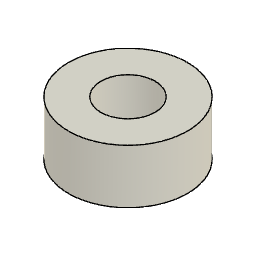
オムニ2024-Complete v4 (Autodesk Fusion 360 archive; units mm, degrees)
design "シリコンチューブ"
Autodesk Fusion 360 part; units mm, degrees
sketch "スケッチ1" plane through (0, 0, 0) normal (0, 0, 1) x (1, 0, 0)
  circle A0 centre (0, 0) radius 5.5
  circle A1 centre (0, 0) radius 2.5
  dimension "d1" = 11
  dimension "d2" = 5
  constraint coincident A0.centre A1.centre
  measures "d1" diameter of A0
  measures "d2" diameter of A1
extrude "押し出し1" add sketch "スケッチ1" along normal blind 5

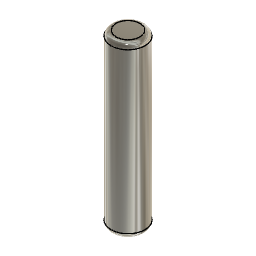
design "棒"
Autodesk Fusion 360 part; units mm, degrees
sketch "スケッチ1" plane through (0, 0, 0) normal (0, 0, 1) x (1, 0, 0)
  circle A0 centre (0, 0) radius 1
  dimension "d1" = 2
  constraint coincident A0.centre origin
  measures "d1" diameter of A0
extrude "押し出し1" add sketch "スケッチ1" along normal blind 10
fillet "フィレット1" radius 0.3 2 edges at (-0.9323, -0.3616, 10) (-0.9323, -0.3616, 0)

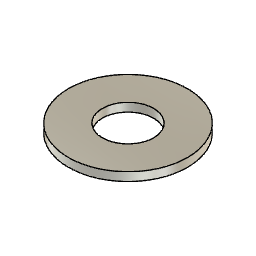
design "ワッシャー　小"
Autodesk Fusion 360 part; units mm, degrees
sketch "スケッチ1" plane through (0, 0, 0) normal (0, 0, 1) x (1, 0, 0)
  circle A0 centre (0, 0) radius 1.5
  circle A1 centre (0, 0) radius 3.5
  dimension "d1" = 3
  dimension "d2" = 7
  constraint coincident A0.centre A1.centre
  measures "d1" diameter of A0
  measures "d2" diameter of A1
extrude "押し出し1" add sketch "スケッチ1" along normal blind 0.5

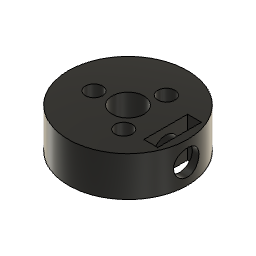
design "オムニ2024-3"
Autodesk Fusion 360 part; units mm, degrees
sketch "スケッチ1" plane through (0, 0, 0) normal (0, 0, 1) x (1, 0, 0)
  circle A0 centre (0, 0) radius 7.5
  dimension "d1" = 15
  constraint coincident A0.centre origin
  measures "d1" diameter of A0
extrude "押し出し1" add sketch "スケッチ1" along normal blind 5
sketch "スケッチ2" plane through (0, 0, 5) normal (0, 0, 1) x (-1, 0, 0)
  circle A0 centre (0, 0) radius 7.5
  circle A1 centre (0, 0) radius 2
  dimension "d4" = 4
  constraint coincident A0.centre A1.centre
  measures "d4" diameter of A1
extrude "押し出し2" cut sketch "スケッチ2" against normal blind 18 contours A1
sketch "スケッチ3" plane through (0, 0, -15) normal (0, 0, 1) x (-1, 0, 0)
  circle A0 centre (-1.3364, -3.4921) radius 1.075
  circle A1 centre (3.6924, 0.5887) radius 1.075
  circle A2 centre (-2.3561, 2.9034) radius 1.075
  circle A3 centre (0, 0) radius 2
  arc A4 (6.9441, -2.8337) -> (7.4957, 0.253) centre (0, 0) ccw
  line L0 (7.4957, 0.253) -> (3.5477, 3.5514)
  arc A5 (3.8294, 4.4336) -> (3.5477, 3.5514) centre (3.8682, 3.9351) ccw
  line L1 (3.8294, 4.4336) -> (5.9261, 4.5969)
  arc A6 (5.9261, 4.5969) -> (3.5288, 6.618) centre (0, 0) ccw
  line L2 (3.5288, 6.618) -> (-1.3018, 4.8481)
  arc A7 (-1.9249, 5.5332) -> (-1.3018, 4.8481) centre (-1.4738, 5.3176) ccw
  line L3 (-1.9249, 5.5332) -> (-1.0179, 7.4306)
  arc A8 (-1.0179, 7.4306) -> (-3.967, 6.365) centre (0, 0) ccw
  line L4 (-3.967, 6.365) -> (-4.8495, 1.2966)
  arc A9 (-5.7543, 1.0996) -> (-4.8495, 1.2966) centre (-5.342, 1.3824) ccw
  line L5 (-5.7543, 1.0996) -> (-6.9441, 2.8337)
  arc A10 (-6.9441, 2.8337) -> (-7.4957, -0.253) centre (0, 0) ccw
  line L6 (-7.4957, -0.253) -> (-3.5477, -3.5514)
  arc A11 (-3.8294, -4.4336) -> (-3.5477, -3.5514) centre (-3.8682, -3.9351) ccw
  line L7 (-3.8294, -4.4336) -> (-5.9261, -4.5969)
  arc A12 (-5.9261, -4.5969) -> (-3.5288, -6.618) centre (0, 0) ccw
  line L8 (-3.5288, -6.618) -> (1.7202, -4.6948)
  arc A13 (1.7202, -4.6948) -> (2.5, -4.3301) centre (0, 0) ccw
  line L9 (2.5, -4.3301) -> (1.0179, -7.4306)
  arc A14 (1.0179, -7.4306) -> (3.967, -6.365) centre (0, 0) ccw
  line L10 (3.967, -6.365) -> (4.8495, -1.2966)
  arc A15 (5.7543, -1.0996) -> (4.8495, -1.2966) centre (5.342, -1.3824) ccw
  line L11 (5.7543, -1.0996) -> (6.9441, -2.8337)
extrude "押し出し3" cut sketch "スケッチ3" along normal blind 28 contours A0 | A1 | A2
sketch "スケッチ4" plane through (0, 0, 0) normal (1, 0, 0) x (0, 1, 0)
  circle A0 centre (0, 2.5) radius 1.6
  dimension "d9" = 3.2
  measures "d9" diameter of A0
extrude "押し出し4" cut sketch "スケッチ4" along normal blind 10
sketch "スケッチ5" plane through (0, 0, 5) normal (0, 0, 1) x (-1, 0, 0)
  circle A0 centre (-1.3364, -3.4921) radius 1.075
  circle A1 centre (3.6924, 0.5887) radius 1.075
  circle A2 centre (-2.3561, 2.9034) radius 1.075
  circle A3 centre (0, 0) radius 2
  circle A4 centre (0, 0) radius 7.5
  line L0 (-4.75, 0) -> (-4.75, 2.75)
  line L1 (-4.75, 2.75) -> (-6.5, 2.75)
  line L2 (-6.5, 2.75) -> (-6.5, 0)
  line L3 (-6.5, -2.75) -> (-6.5, 0)
  line L4 (-4.75, 0) -> (-4.75, -2.75)
  line L5 (-4.75, -2.75) -> (-6.5, -2.75)
  dimension "d12" = 1.75
  dimension "d13" = 2.75
  constraint vertical L0
  constraint horizontal L1
  constraint vertical L2
  measures "d12" distance of L2.end L0.start
  measures "d13" distance of L2.end L1.end
extrude "押し出し5" cut sketch "スケッチ5" against normal blind 9 contours L0 L1 L2 L3 L4 L5

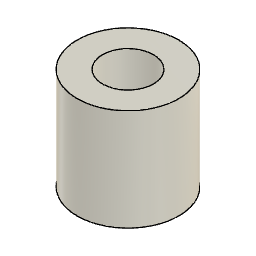
design "プラスチックスペーサー"
Autodesk Fusion 360 part; units mm, degrees
sketch "スケッチ1" plane through (0, 0, 0) normal (0, 0, 1) x (1, 0, 0)
  circle A0 centre (0, 0) radius 2.5
  circle A1 centre (0, 0) radius 1.25
  dimension "d1" = 5
  dimension "d2" = 2.5
  constraint coincident A0.centre A1.centre
  constraint concentric A0 A1
  measures "d1" diameter of A0
  measures "d2" diameter of A1
extrude "押し出し1" add sketch "スケッチ1" along normal blind 5

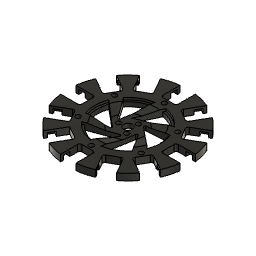
design "オムニ2024-1"
Autodesk Fusion 360 part; units mm, degrees
sketch "スケッチ2" plane through (0, 0, 0) normal (0, 0, 1) x (1, 0, 0)
  circle A0 centre (0, 0) radius 27.5
  line L0 (-3.5, 18.5) -> (3.5, 18.5)
  line L1 (3.5, 18.5) -> (3.5, 30.5)
  line L2 (3.5, 30.5) -> (-3.5, 30.5)
  line L3 (-3.5, 30.5) -> (-3.5, 18.5)
  line L4 (-18.2811, 24.6638) -> (-12.2811, 14.2715)
  line L5 (-6.2189, 17.7715) -> (-12.2189, 28.1638)
  line L6 (-12.2811, 14.2715) -> (-6.2189, 17.7715)
  line L7 (-12.2189, 28.1638) -> (-18.2811, 24.6638)
  line L8 (-28.1638, 12.2189) -> (-17.7715, 6.2189)
  line L9 (-14.2715, 12.2811) -> (-24.6638, 18.2811)
  line L10 (-17.7715, 6.2189) -> (-14.2715, 12.2811)
  line L11 (-24.6638, 18.2811) -> (-28.1638, 12.2189)
  line L12 (-30.5, -3.5) -> (-18.5, -3.5)
  line L13 (-18.5, 3.5) -> (-30.5, 3.5)
  line L14 (-18.5, -3.5) -> (-18.5, 3.5)
  line L15 (-30.5, 3.5) -> (-30.5, -3.5)
  line L16 (-24.6638, -18.2811) -> (-14.2715, -12.2811)
  line L17 (-17.7715, -6.2189) -> (-28.1638, -12.2189)
  line L18 (-14.2715, -12.2811) -> (-17.7715, -6.2189)
  line L19 (-28.1638, -12.2189) -> (-24.6638, -18.2811)
  line L20 (-12.2189, -28.1638) -> (-6.2189, -17.7715)
  line L21 (-12.2811, -14.2715) -> (-18.2811, -24.6638)
  line L22 (-6.2189, -17.7715) -> (-12.2811, -14.2715)
  line L23 (-18.2811, -24.6638) -> (-12.2189, -28.1638)
  line L24 (3.5, -30.5) -> (3.5, -18.5)
  line L25 (-3.5, -18.5) -> (-3.5, -30.5)
  line L26 (3.5, -18.5) -> (-3.5, -18.5)
  line L27 (-3.5, -30.5) -> (3.5, -30.5)
  line L28 (18.2811, -24.6638) -> (12.2811, -14.2715)
  line L29 (6.2189, -17.7715) -> (12.2189, -28.1638)
  line L30 (12.2811, -14.2715) -> (6.2189, -17.7715)
  line L31 (12.2189, -28.1638) -> (18.2811, -24.6638)
  line L32 (28.1638, -12.2189) -> (17.7715, -6.2189)
  line L33 (14.2715, -12.2811) -> (24.6638, -18.2811)
  line L34 (17.7715, -6.2189) -> (14.2715, -12.2811)
  line L35 (24.6638, -18.2811) -> (28.1638, -12.2189)
  line L36 (30.5, 3.5) -> (18.5, 3.5)
  line L37 (18.5, -3.5) -> (30.5, -3.5)
  line L38 (18.5, 3.5) -> (18.5, -3.5)
  line L39 (30.5, -3.5) -> (30.5, 3.5)
  line L40 (24.6638, 18.2811) -> (14.2715, 12.2811)
  line L41 (17.7715, 6.2189) -> (28.1638, 12.2189)
  line L42 (14.2715, 12.2811) -> (17.7715, 6.2189)
  line L43 (28.1638, 12.2189) -> (24.6638, 18.2811)
  line L44 (12.2189, 28.1638) -> (6.2189, 17.7715)
  line L45 (12.2811, 14.2715) -> (18.2811, 24.6638)
  line L46 (6.2189, 17.7715) -> (12.2811, 14.2715)
  line L47 (18.2811, 24.6638) -> (12.2189, 28.1638)
  dimension "d2" = 55
  dimension "d4" = 360
  constraint coincident A0.centre origin
  constraint horizontal L0
  constraint vertical L1
  constraint horizontal L2
  constraint vertical L3
  measures "d2" diameter of A0
extrude "押し出し1" add sketch "スケッチ2" along normal blind 3 contours A0 L0 L1 L3 L4 L5 L6 L8 L9 L10 L12 L13 L14 L16 L17 L18 L20 L21 L22 L24 L25 L26 L28 L29 L30 L32 L33 L34 L36 L37 L38 L40 L41 L42 L44 L45 L46
sketch "スケッチ3" plane through (0, 0, 3) normal (0, 0, 1) x (-1, 0, 0)
  arc A0 (-10.6071, -25.372) -> (-3.5, -27.2764) centre (0, 0) ccw
  line L0 (-3.5, -27.2764) -> (-3.5, -18.5)
  line L1 (-3.5, -18.5) -> (3.5, -18.5)
  line L2 (3.5, -18.5) -> (3.5, -27.2764)
  arc A1 (3.5, -27.2764) -> (10.6071, -25.372) centre (0, 0) ccw
  line L3 (10.6071, -25.372) -> (6.2189, -17.7715)
  line L4 (6.2189, -17.7715) -> (12.2811, -14.2715)
  line L5 (12.2811, -14.2715) -> (16.6693, -21.872)
  arc A2 (16.6693, -21.872) -> (21.872, -16.6693) centre (0, 0) ccw
  line L6 (21.872, -16.6693) -> (14.2715, -12.2811)
  line L7 (14.2715, -12.2811) -> (17.7715, -6.2189)
  line L8 (17.7715, -6.2189) -> (25.372, -10.6071)
  arc A3 (25.372, -10.6071) -> (27.2764, -3.5) centre (0, 0) ccw
  line L9 (27.2764, -3.5) -> (18.5, -3.5)
  line L10 (18.5, -3.5) -> (18.5, 3.5)
  line L11 (18.5, 3.5) -> (27.2764, 3.5)
  arc A4 (27.2764, 3.5) -> (25.372, 10.6071) centre (0, 0) ccw
  line L12 (25.372, 10.6071) -> (17.7715, 6.2189)
  line L13 (17.7715, 6.2189) -> (14.2715, 12.2811)
  line L14 (14.2715, 12.2811) -> (21.872, 16.6693)
  arc A5 (21.872, 16.6693) -> (16.6693, 21.872) centre (0, 0) ccw
  line L15 (16.6693, 21.872) -> (12.2811, 14.2715)
  line L16 (12.2811, 14.2715) -> (6.2189, 17.7715)
  line L17 (6.2189, 17.7715) -> (10.6071, 25.372)
  arc A6 (10.6071, 25.372) -> (3.5, 27.2764) centre (0, 0) ccw
  line L18 (3.5, 27.2764) -> (3.5, 18.5)
  line L19 (3.5, 18.5) -> (-3.5, 18.5)
  line L20 (-3.5, 18.5) -> (-3.5, 27.2764)
  arc A7 (-3.5, 27.2764) -> (-10.6071, 25.372) centre (0, 0) ccw
  line L21 (-10.6071, 25.372) -> (-6.2189, 17.7715)
  line L22 (-6.2189, 17.7715) -> (-12.2811, 14.2715)
  line L23 (-12.2811, 14.2715) -> (-16.6693, 21.872)
  arc A8 (-16.6693, 21.872) -> (-21.872, 16.6693) centre (0, 0) ccw
  line L24 (-21.872, 16.6693) -> (-14.2715, 12.2811)
  line L25 (-14.2715, 12.2811) -> (-17.7715, 6.2189)
  line L26 (-17.7715, 6.2189) -> (-25.372, 10.6071)
  arc A9 (-25.372, 10.6071) -> (-27.2764, 3.5) centre (0, 0) ccw
  line L27 (-27.2764, 3.5) -> (-18.5, 3.5)
  line L28 (-18.5, 3.5) -> (-18.5, -3.5)
  line L29 (-18.5, -3.5) -> (-27.2764, -3.5)
  arc A10 (-27.2764, -3.5) -> (-25.372, -10.6071) centre (0, 0) ccw
  line L30 (-25.372, -10.6071) -> (-17.7715, -6.2189)
  line L31 (-17.7715, -6.2189) -> (-14.2715, -12.2811)
  line L32 (-14.2715, -12.2811) -> (-21.872, -16.6693)
  arc A11 (-21.872, -16.6693) -> (-16.6693, -21.872) centre (0, 0) ccw
  line L33 (-16.6693, -21.872) -> (-12.2811, -14.2715)
  line L34 (-12.2811, -14.2715) -> (-6.2189, -17.7715)
  line L35 (-6.2189, -17.7715) -> (-10.6071, -25.372)
  circle A12 centre (0, 0) radius 15
  circle A13 centre (0, 0) radius 2
  circle A14 centre (0, 0) radius 5
  line L36 (2.5, -14.7902) -> (4.9259, -0.8577)
  line L37 (-2.5, -14.7902) -> (2.5, -4.3301)
  line L38 (14.0587, -5.23) -> (3.2057, 3.8371)
  line L39 (11.5587, -9.5602) -> (5, 0)
  line L40 (11.5587, 9.5602) -> (-1.7202, 4.6948)
  line L41 (14.0587, 5.23) -> (2.5, 4.3301)
  line L42 (-2.5, 14.7902) -> (-4.9259, 0.8577)
  line L43 (2.5, 14.7902) -> (-2.5, 4.3301)
  line L44 (-14.0587, 5.23) -> (-3.2057, -3.8371)
  line L45 (-11.5587, 9.5602) -> (-5, 0)
  line L46 (-11.5587, -9.5602) -> (1.7202, -4.6948)
  line L47 (-14.0587, -5.23) -> (-2.5, -4.3301)
  dimension "d8" = 360
  constraint coincident A0.centre A1.centre
  constraint concentric A12 A14
  constraint coincident A12 L36.start
  constraint coincident A14 L36.end
  constraint tangent A14 L36
  constraint coincident A12 L37.start
  constraint coincident A14 L37.end
extrude "押し出し2" cut sketch "スケッチ3" against normal blind 30 contours A12 A14 L38 L41 | A12 A14 L40 L43 | A12 A14 L36 L39 | A12 A14 L42 L45 | A12 A14 L37 L46 | A12 A14 L44 L47 | A13
sketch "スケッチ4" plane through (0, 0, 0) normal (0, 1, 0) x (1, 0, 0)
  line L0 (0, -6) -> (0, -2)
  line L1 (0, -2) -> (10, -3)
  line L2 (10, -3) -> (10, -7)
  line L3 (10, -7) -> (0, -6)
  constraint vertical L0
  constraint parallel L0 L2
sketch "スケッチ5" plane through (0, 0, 0) normal (0, 0, 1) x (1, 0, 0)
  circle A0 centre (0, 0) radius 15
  circle A1 centre (0, 0) radius 14
  constraint coincident A0.centre A1.centre
extrude "押し出し3" add sketch "スケッチ5" along normal blind 2
sketch "スケッチ6" plane through (0, 0, 0) normal (0, 0, -1) x (1, 0, 0)
  line L0 (-13.0187, 5.1491) -> (-2.5, 4.3301)
  arc A0 (-2.5, 4.3301) -> (-3.2057, 3.8371) centre (0, 0) ccw
  line L1 (-3.2057, 3.8371) -> (-13.241, -4.5469)
  arc A1 (-13.0187, 5.1491) -> (-13.241, -4.5469) centre (0, 0) ccw
  line L2 (-10.9686, -8.7) -> (-5, 0)
  arc A2 (-5, 0) -> (-4.9259, -0.8577) centre (0, 0) ccw
  line L3 (-4.9259, -0.8577) -> (-2.6828, -13.7406)
  arc A3 (-10.9686, -8.7) -> (-2.6828, -13.7406) centre (0, 0) ccw
  line L4 (2.0501, -13.8491) -> (-2.5, -4.3301)
  arc A4 (-2.5, -4.3301) -> (-1.7202, -4.6948) centre (0, 0) ccw
  line L5 (-1.7202, -4.6948) -> (10.5583, -9.1936)
  arc A5 (2.0501, -13.8491) -> (10.5583, -9.1936) centre (0, 0) ccw
  arc A6 (-2.0501, 13.8491) -> (-10.5583, 9.1936) centre (0, 0) ccw
  line L6 (-2.0501, 13.8491) -> (2.5, 4.3301)
  arc A7 (2.5, 4.3301) -> (1.7202, 4.6948) centre (0, 0) ccw
  line L7 (1.7202, 4.6948) -> (-10.5583, 9.1936)
  arc A8 (10.9686, 8.7) -> (2.6828, 13.7406) centre (0, 0) ccw
  line L8 (10.9686, 8.7) -> (5, 0)
  arc A9 (5, 0) -> (4.9259, 0.8577) centre (0, 0) ccw
  line L9 (4.9259, 0.8577) -> (2.6828, 13.7406)
  circle A10 centre (0, 0) radius 2
  arc A11 (13.0187, -5.1491) -> (13.241, 4.5469) centre (0, 0) ccw
  line L10 (13.0187, -5.1491) -> (2.5, -4.3301)
  arc A12 (2.5, -4.3301) -> (3.2057, -3.8371) centre (0, 0) ccw
  line L11 (3.2057, -3.8371) -> (13.241, 4.5469)
  arc A13 (3.5, -27.2764) -> (10.6071, -25.372) centre (0, 0) ccw
  line L12 (10.6071, -25.372) -> (6.2189, -17.7715)
  line L13 (6.2189, -17.7715) -> (12.2811, -14.2715)
  line L14 (12.2811, -14.2715) -> (16.6693, -21.872)
  arc A14 (16.6693, -21.872) -> (21.872, -16.6693) centre (0, 0) ccw
  line L15 (21.872, -16.6693) -> (14.2715, -12.2811)
  line L16 (14.2715, -12.2811) -> (17.7715, -6.2189)
  line L17 (17.7715, -6.2189) -> (25.372, -10.6071)
  arc A15 (25.372, -10.6071) -> (27.2764, -3.5) centre (0, 0) ccw
  line L18 (27.2764, -3.5) -> (18.5, -3.5)
  line L19 (18.5, -3.5) -> (18.5, 3.5)
  line L20 (18.5, 3.5) -> (27.2764, 3.5)
  arc A16 (27.2764, 3.5) -> (25.372, 10.6071) centre (0, 0) ccw
  line L21 (25.372, 10.6071) -> (17.7715, 6.2189)
  line L22 (17.7715, 6.2189) -> (14.2715, 12.2811)
  line L23 (14.2715, 12.2811) -> (21.872, 16.6693)
  arc A17 (21.872, 16.6693) -> (16.6693, 21.872) centre (0, 0) ccw
  line L24 (16.6693, 21.872) -> (12.2811, 14.2715)
  line L25 (12.2811, 14.2715) -> (6.2189, 17.7715)
  line L26 (6.2189, 17.7715) -> (10.6071, 25.372)
  arc A18 (10.6071, 25.372) -> (3.5, 27.2764) centre (0, 0) ccw
  line L27 (3.5, 27.2764) -> (3.5, 18.5)
  line L28 (3.5, 18.5) -> (-3.5, 18.5)
  line L29 (-3.5, 18.5) -> (-3.5, 27.2764)
  arc A19 (-3.5, 27.2764) -> (-10.6071, 25.372) centre (0, 0) ccw
  line L30 (-10.6071, 25.372) -> (-6.2189, 17.7715)
  line L31 (-6.2189, 17.7715) -> (-12.2811, 14.2715)
  line L32 (-12.2811, 14.2715) -> (-16.6693, 21.872)
  arc A20 (-16.6693, 21.872) -> (-21.872, 16.6693) centre (0, 0) ccw
  line L33 (-21.872, 16.6693) -> (-14.2715, 12.2811)
  line L34 (-14.2715, 12.2811) -> (-17.7715, 6.2189)
  line L35 (-17.7715, 6.2189) -> (-25.372, 10.6071)
  arc A21 (-25.372, 10.6071) -> (-27.2764, 3.5) centre (0, 0) ccw
  line L36 (-27.2764, 3.5) -> (-18.5, 3.5)
  line L37 (-18.5, 3.5) -> (-18.5, -3.5)
  line L38 (-18.5, -3.5) -> (-27.2764, -3.5)
  arc A22 (-27.2764, -3.5) -> (-25.372, -10.6071) centre (0, 0) ccw
  line L39 (-25.372, -10.6071) -> (-17.7715, -6.2189)
  line L40 (-17.7715, -6.2189) -> (-14.2715, -12.2811)
  line L41 (-14.2715, -12.2811) -> (-21.872, -16.6693)
  arc A23 (-21.872, -16.6693) -> (-16.6693, -21.872) centre (0, 0) ccw
  line L42 (-16.6693, -21.872) -> (-12.2811, -14.2715)
  line L43 (-12.2811, -14.2715) -> (-6.2189, -17.7715)
  line L44 (-6.2189, -17.7715) -> (-10.6071, -25.372)
  arc A24 (-10.6071, -25.372) -> (-3.5, -27.2764) centre (0, 0) ccw
  line L45 (-3.5, -27.2764) -> (-3.5, -18.5)
  line L46 (-3.5, -18.5) -> (3.5, -18.5)
  line L47 (3.5, -18.5) -> (3.5, -27.2764)
  line L48 (5.4, -26) -> (0, -26)
  line L49 (0, -23) -> (5.4, -23)
  line L50 (5.4, -23) -> (5.4, -26)
  line L51 (0, -23) -> (-5.4, -23)
  line L52 (-5.4, -23) -> (-5.4, -26)
  line L53 (-5.4, -26) -> (0, -26)
  line L54 (11.5, -19.9186) -> (6.8235, -22.6186)
  line L55 (6.8235, -22.6186) -> (8.3235, -25.2167)
  line L56 (8.3235, -25.2167) -> (13, -22.5167)
  line L57 (17.6765, -19.8167) -> (13, -22.5167)
  line L58 (11.5, -19.9186) -> (16.1765, -17.2186)
  line L59 (16.1765, -17.2186) -> (17.6765, -19.8167)
  line L60 (19.9186, -11.5) -> (17.2186, -16.1765)
  line L61 (17.2186, -16.1765) -> (19.8167, -17.6765)
  line L62 (19.8167, -17.6765) -> (22.5167, -13)
  line L63 (25.2167, -8.3235) -> (22.5167, -13)
  line L64 (19.9186, -11.5) -> (22.6186, -6.8235)
  line L65 (22.6186, -6.8235) -> (25.2167, -8.3235)
  line L66 (23, 0) -> (23, -5.4)
  line L67 (23, -5.4) -> (26, -5.4)
  line L68 (26, -5.4) -> (26, 0)
  line L69 (26, 5.4) -> (26, 0)
  line L70 (23, 0) -> (23, 5.4)
  line L71 (23, 5.4) -> (26, 5.4)
  line L72 (19.9186, 11.5) -> (22.6186, 6.8235)
  line L73 (22.6186, 6.8235) -> (25.2167, 8.3235)
  line L74 (25.2167, 8.3235) -> (22.5167, 13)
  line L75 (19.8167, 17.6765) -> (22.5167, 13)
  line L76 (19.9186, 11.5) -> (17.2186, 16.1765)
  line L77 (17.2186, 16.1765) -> (19.8167, 17.6765)
  line L78 (11.5, 19.9186) -> (16.1765, 17.2186)
  line L79 (16.1765, 17.2186) -> (17.6765, 19.8167)
  line L80 (17.6765, 19.8167) -> (13, 22.5167)
  line L81 (8.3235, 25.2167) -> (13, 22.5167)
  line L82 (11.5, 19.9186) -> (6.8235, 22.6186)
  line L83 (6.8235, 22.6186) -> (8.3235, 25.2167)
  line L84 (0, 23) -> (5.4, 23)
  line L85 (5.4, 23) -> (5.4, 26)
  line L86 (5.4, 26) -> (0, 26)
  line L87 (-5.4, 26) -> (0, 26)
  line L88 (0, 23) -> (-5.4, 23)
  line L89 (-5.4, 23) -> (-5.4, 26)
  line L90 (-11.5, 19.9186) -> (-6.8235, 22.6186)
  line L91 (-6.8235, 22.6186) -> (-8.3235, 25.2167)
  line L92 (-8.3235, 25.2167) -> (-13, 22.5167)
  line L93 (-17.6765, 19.8167) -> (-13, 22.5167)
  line L94 (-11.5, 19.9186) -> (-16.1765, 17.2186)
  line L95 (-16.1765, 17.2186) -> (-17.6765, 19.8167)
  line L96 (-19.9186, 11.5) -> (-17.2186, 16.1765)
  line L97 (-17.2186, 16.1765) -> (-19.8167, 17.6765)
  line L98 (-19.8167, 17.6765) -> (-22.5167, 13)
  line L99 (-25.2167, 8.3235) -> (-22.5167, 13)
  line L100 (-19.9186, 11.5) -> (-22.6186, 6.8235)
  line L101 (-22.6186, 6.8235) -> (-25.2167, 8.3235)
  line L102 (-23, 0) -> (-23, 5.4)
  line L103 (-23, 5.4) -> (-26, 5.4)
  line L104 (-26, 5.4) -> (-26, 0)
  line L105 (-26, -5.4) -> (-26, 0)
  line L106 (-23, 0) -> (-23, -5.4)
  line L107 (-23, -5.4) -> (-26, -5.4)
  line L108 (-19.9186, -11.5) -> (-22.6186, -6.8235)
  line L109 (-22.6186, -6.8235) -> (-25.2167, -8.3235)
  line L110 (-25.2167, -8.3235) -> (-22.5167, -13)
  line L111 (-19.8167, -17.6765) -> (-22.5167, -13)
  line L112 (-19.9186, -11.5) -> (-17.2186, -16.1765)
  line L113 (-17.2186, -16.1765) -> (-19.8167, -17.6765)
  line L114 (-11.5, -19.9186) -> (-16.1765, -17.2186)
  line L115 (-16.1765, -17.2186) -> (-17.6765, -19.8167)
  line L116 (-17.6765, -19.8167) -> (-13, -22.5167)
  line L117 (-8.3235, -25.2167) -> (-13, -22.5167)
  line L118 (-11.5, -19.9186) -> (-6.8235, -22.6186)
  line L119 (-6.8235, -22.6186) -> (-8.3235, -25.2167)
  dimension "d15" = 360
  constraint horizontal L48
  constraint horizontal L49
  constraint vertical L50
extrude "押し出し4" cut sketch "スケッチ6" against normal blind 2 contours L47 L48 L49 L50 | L12 L54 L55 L56 | L45 L51 L52 L53 | L14 L57 L58 L59 | L44 L117 L118 L119 | L15 L60 L61 L62 | L42 L114 L115 L116 | L17 L63 L64 L65 | L41 L111 L112 L113 | L18 L66 L67 L68 | L39 L108 L109 L110 | L20 L69 L70 L71 | L38 L105 L106 L107 | L21 L72 L73 L74 | L36 L102 L103 L104 | L23 L75 L76 L77 | L35 L99 L100 L101 | L24 L78 L79 L80 | L33 L96 L97 L98 | L26 L81 L82 L83 | L32 L93 L94 L95 | L27 L84 L85 L86 | L30 L90 L91 L92 | L29 L87 L88 L89
sketch "スケッチ7" plane through (0, 0, 3) normal (0, 0, 1) x (-1, 0, 0)
  line L0 (-2.5, 4.3301) -> (2.5, 14.7902)
  arc A0 (11.5587, 9.5602) -> (2.5, 14.7902) centre (0, 0) ccw
  line L1 (11.5587, 9.5602) -> (-1.7202, 4.6948)
  arc A1 (-1.7202, 4.6948) -> (-2.5, 4.3301) centre (0, 0) ccw
  line L2 (5, 0) -> (11.5587, -9.5602)
  arc A2 (2.5, -14.7902) -> (11.5587, -9.5602) centre (0, 0) ccw
  line L3 (2.5, -14.7902) -> (4.9259, -0.8577)
  arc A3 (4.9259, -0.8577) -> (5, 0) centre (0, 0) ccw
  line L4 (-5, 0) -> (-11.5587, 9.5602)
  arc A4 (-2.5, 14.7902) -> (-11.5587, 9.5602) centre (0, 0) ccw
  line L5 (-2.5, 14.7902) -> (-4.9259, 0.8577)
  arc A5 (-4.9259, 0.8577) -> (-5, 0) centre (0, 0) ccw
  line L6 (2.5, 4.3301) -> (14.0587, 5.23)
  arc A6 (14.0587, -5.23) -> (14.0587, 5.23) centre (0, 0) ccw
  line L7 (14.0587, -5.23) -> (3.2057, 3.8371)
  arc A7 (3.2057, 3.8371) -> (2.5, 4.3301) centre (0, 0) ccw
  arc A8 (1.7202, -4.6948) -> (2.5, -4.3301) centre (0, 0) ccw
  line L8 (2.5, -4.3301) -> (-2.5, -14.7902)
  arc A9 (-11.5587, -9.5602) -> (-2.5, -14.7902) centre (0, 0) ccw
  line L9 (-11.5587, -9.5602) -> (1.7202, -4.6948)
  line L10 (-2.5, -4.3301) -> (-14.0587, -5.23)
  arc A10 (-14.0587, 5.23) -> (-14.0587, -5.23) centre (0, 0) ccw
  line L11 (-14.0587, 5.23) -> (-3.2057, -3.8371)
  arc A11 (-3.2057, -3.8371) -> (-2.5, -4.3301) centre (0, 0) ccw
  circle A12 centre (0, 0) radius 2
  arc A13 (-10.6071, -25.372) -> (-3.5, -27.2764) centre (0, 0) ccw
  line L12 (-3.5, -27.2764) -> (-3.5, -18.5)
  line L13 (-3.5, -18.5) -> (3.5, -18.5)
  line L14 (3.5, -18.5) -> (3.5, -27.2764)
  arc A14 (3.5, -27.2764) -> (10.6071, -25.372) centre (0, 0) ccw
  line L15 (10.6071, -25.372) -> (6.2189, -17.7715)
  line L16 (6.2189, -17.7715) -> (12.2811, -14.2715)
  line L17 (12.2811, -14.2715) -> (16.6693, -21.872)
  arc A15 (16.6693, -21.872) -> (21.872, -16.6693) centre (0, 0) ccw
  line L18 (21.872, -16.6693) -> (14.2715, -12.2811)
  line L19 (14.2715, -12.2811) -> (17.7715, -6.2189)
  line L20 (17.7715, -6.2189) -> (25.372, -10.6071)
  arc A16 (25.372, -10.6071) -> (27.2764, -3.5) centre (0, 0) ccw
  line L21 (27.2764, -3.5) -> (18.5, -3.5)
  line L22 (18.5, -3.5) -> (18.5, 3.5)
  line L23 (18.5, 3.5) -> (27.2764, 3.5)
  arc A17 (27.2764, 3.5) -> (25.372, 10.6071) centre (0, 0) ccw
  line L24 (25.372, 10.6071) -> (17.7715, 6.2189)
  line L25 (17.7715, 6.2189) -> (14.2715, 12.2811)
  line L26 (14.2715, 12.2811) -> (21.872, 16.6693)
  arc A18 (21.872, 16.6693) -> (16.6693, 21.872) centre (0, 0) ccw
  line L27 (16.6693, 21.872) -> (12.2811, 14.2715)
  line L28 (12.2811, 14.2715) -> (6.2189, 17.7715)
  line L29 (6.2189, 17.7715) -> (10.6071, 25.372)
  arc A19 (10.6071, 25.372) -> (3.5, 27.2764) centre (0, 0) ccw
  line L30 (3.5, 27.2764) -> (3.5, 18.5)
  line L31 (3.5, 18.5) -> (-3.5, 18.5)
  line L32 (-3.5, 18.5) -> (-3.5, 27.2764)
  arc A20 (-3.5, 27.2764) -> (-10.6071, 25.372) centre (0, 0) ccw
  line L33 (-10.6071, 25.372) -> (-6.2189, 17.7715)
  line L34 (-6.2189, 17.7715) -> (-12.2811, 14.2715)
  line L35 (-12.2811, 14.2715) -> (-16.6693, 21.872)
  arc A21 (-16.6693, 21.872) -> (-21.872, 16.6693) centre (0, 0) ccw
  line L36 (-21.872, 16.6693) -> (-14.2715, 12.2811)
  line L37 (-14.2715, 12.2811) -> (-17.7715, 6.2189)
  line L38 (-17.7715, 6.2189) -> (-25.372, 10.6071)
  arc A22 (-25.372, 10.6071) -> (-27.2764, 3.5) centre (0, 0) ccw
  line L39 (-27.2764, 3.5) -> (-18.5, 3.5)
  line L40 (-18.5, 3.5) -> (-18.5, -3.5)
  line L41 (-18.5, -3.5) -> (-27.2764, -3.5)
  arc A23 (-27.2764, -3.5) -> (-25.372, -10.6071) centre (0, 0) ccw
  line L42 (-25.372, -10.6071) -> (-17.7715, -6.2189)
  line L43 (-17.7715, -6.2189) -> (-14.2715, -12.2811)
  line L44 (-14.2715, -12.2811) -> (-21.872, -16.6693)
  arc A24 (-21.872, -16.6693) -> (-16.6693, -21.872) centre (0, 0) ccw
  line L45 (-16.6693, -21.872) -> (-12.2811, -14.2715)
  line L46 (-12.2811, -14.2715) -> (-6.2189, -17.7715)
  line L47 (-6.2189, -17.7715) -> (-10.6071, -25.372)
  circle A25 centre (0, 0) radius 7.5
  dimension "d18" = 15
  constraint concentric A0 A25
  measures "d18" diameter of A25
extrude "押し出し5" cut sketch "スケッチ7" against normal blind 1 contours L0 L1 A1 L2 L3 A3 L4 L5 A5 L6 L7 A7 A8 L8 L9 L10 L11 A11 A25
sketch "スケッチ8" plane through (0, 0, 0) normal (0, 1, 0) x (1, 0, 0)
  line L0 (0, -10) -> (-7.5, -10)
  line L1 (0, -10) -> (0, -2)
  line L2 (0, -2) -> (-7.5, -2)
  line L3 (-7.5, -2) -> (-13, -3)
  line L4 (-13, -3) -> (-8, -10)
  line L5 (-8, -10) -> (-7.5, -10)
  dimension "d21" = 7.5
  dimension "d22" = 7.5
  constraint horizontal L0
  constraint perpendicular L0 L1
  constraint perpendicular L1 L2
  constraint parallel L0 L5
  measures "d21" distance of L0.start L0.end
  measures "d22" distance of L1.end L2.end
revolve "回転2" cut sketch "スケッチ8" angle 360 about axis through (0, 0, 10) along (0, 0, -1)
fillet "フィレット1" radius 0.5 5 edges at (2.5, 4.3301, 1) (-5, 0, 1) (-2.5, -4.3301, 1) (2.5, -4.3301, 1) (5, 0, 1)
fillet "フィレット2" radius 1 23 edges at (-12.2811, 14.2715, 1.5) (-6.2189, 17.7715, 1.5) (-3.5, 18.5, 1.5) (3.5, 18.5, 1.5) (6.2189, 17.7715, 1.5) (12.2811, 14.2715, 1.5) (14.2715, 12.2811, 1.5) (17.7715, 6.2189, 1.5) (18.5, 3.5, 1.5) (18.5, -3.5, 1.5) (17.7715, -6.2189, 1.5) (14.2715, -12.2811, 1.5) (12.2811, -14.2715, 1.5) (6.2189, -17.7715, 1.5) (3.5, -18.5, 1.5) (-3.5, -18.5, 1.5) (-6.2189, -17.7715, 1.5) (-14.2715, -12.2811, 1.5) (-17.7715, -6.2189, 1.5) (-18.5, -3.5, 1.5) (-18.5, 3.5, 1.5) (-17.7715, 6.2189, 1.5) (-14.2715, 12.2811, 1.5)
sketch "スケッチ9" plane through (0, 0, 2) normal (0, 0, 1) x (-1, 0, 0)
  circle A0 centre (0, 0) radius 2
  arc A1 (6.9441, -2.8337) -> (7.4957, 0.253) centre (0, 0) ccw
  line L0 (7.4957, 0.253) -> (3.5477, 3.5514)
  arc A2 (3.8294, 4.4336) -> (3.5477, 3.5514) centre (3.8682, 3.9351) ccw
  line L1 (3.8294, 4.4336) -> (5.9261, 4.5969)
  arc A3 (5.9261, 4.5969) -> (3.5288, 6.618) centre (0, 0) ccw
  line L2 (3.5288, 6.618) -> (-1.3018, 4.8481)
  arc A4 (-1.9249, 5.5332) -> (-1.3018, 4.8481) centre (-1.4738, 5.3176) ccw
  line L3 (-1.9249, 5.5332) -> (-1.0179, 7.4306)
  arc A5 (-1.0179, 7.4306) -> (-3.967, 6.365) centre (0, 0) ccw
  line L4 (-3.967, 6.365) -> (-4.8495, 1.2966)
  arc A6 (-5.7543, 1.0996) -> (-4.8495, 1.2966) centre (-5.342, 1.3824) ccw
  line L5 (-5.7543, 1.0996) -> (-6.9441, 2.8337)
  arc A7 (-6.9441, 2.8337) -> (-7.4957, -0.253) centre (0, 0) ccw
  line L6 (-7.4957, -0.253) -> (-3.5477, -3.5514)
  arc A8 (-3.8294, -4.4336) -> (-3.5477, -3.5514) centre (-3.8682, -3.9351) ccw
  line L7 (-3.8294, -4.4336) -> (-5.9261, -4.5969)
  arc A9 (-5.9261, -4.5969) -> (-3.5288, -6.618) centre (0, 0) ccw
  line L8 (-3.5288, -6.618) -> (1.7202, -4.6948)
  arc A10 (1.7202, -4.6948) -> (2.5, -4.3301) centre (0, 0) ccw
  line L9 (2.5, -4.3301) -> (1.0179, -7.4306)
  arc A11 (1.0179, -7.4306) -> (3.967, -6.365) centre (0, 0) ccw
  line L10 (3.967, -6.365) -> (4.8495, -1.2966)
  arc A12 (5.7543, -1.0996) -> (4.8495, -1.2966) centre (5.342, -1.3824) ccw
  line L11 (5.7543, -1.0996) -> (6.9441, -2.8337)
  circle A13 centre (-1.3364, -3.4921) radius 1.075
  circle A14 centre (3.6924, 0.5887) radius 1.075
  circle A15 centre (-2.3561, 2.9034) radius 1.075
  dimension "d28" = 2.15
  dimension "d30" = 360
  measures "d28" diameter of A13
extrude "押し出し6" cut sketch "スケッチ9" against normal blind 3 contours A13 | A14 | A15
sketch "スケッチ10" plane through (0, 0, 3) normal (0, 0, 1) x (-1, 0, 0)
  arc A0 (10.3744, -7.834) -> (12.4148, -3.8566) centre (0, 0) ccw
  line L0 (10.3744, -7.834) -> (11.5587, -9.5602)
  arc A1 (2.5, -14.7902) -> (11.5587, -9.5602) centre (0, 0) ccw
  line L1 (2.5, -14.7902) -> (2.8675, -12.6798)
  arc A2 (-1.5972, -12.9015) -> (2.8675, -12.6798) centre (0, 0) ccw
  line L2 (-1.5972, -12.9015) -> (-2.5, -14.7902)
  arc A3 (-11.5587, -9.5602) -> (-2.5, -14.7902) centre (0, 0) ccw
  line L3 (-11.5587, -9.5602) -> (-9.5473, -8.8232)
  arc A4 (-11.9716, -5.0675) -> (-9.5473, -8.8232) centre (0, 0) ccw
  line L4 (-11.9716, -5.0675) -> (-14.0587, -5.23)
  arc A5 (-14.0587, 5.23) -> (-14.0587, -5.23) centre (0, 0) ccw
  line L5 (-14.0587, 5.23) -> (-12.4148, 3.8566)
  arc A6 (-10.3744, 7.834) -> (-12.4148, 3.8566) centre (0, 0) ccw
  line L6 (-10.3744, 7.834) -> (-11.5587, 9.5602)
  arc A7 (-2.5, 14.7902) -> (-11.5587, 9.5602) centre (0, 0) ccw
  line L7 (-2.5, 14.7902) -> (-2.8675, 12.6798)
  arc A8 (1.5972, 12.9015) -> (-2.8675, 12.6798) centre (0, 0) ccw
  line L8 (1.5972, 12.9015) -> (2.5, 14.7902)
  arc A9 (11.5587, 9.5602) -> (2.5, 14.7902) centre (0, 0) ccw
  line L9 (11.5587, 9.5602) -> (9.5473, 8.8232)
  arc A10 (11.9716, 5.0675) -> (9.5473, 8.8232) centre (0, 0) ccw
  line L10 (11.9716, 5.0675) -> (14.0587, 5.23)
  arc A11 (14.0587, -5.23) -> (14.0587, 5.23) centre (0, 0) ccw
  line L11 (14.0587, -5.23) -> (12.4148, -3.8566)
  arc A12 (-10.6071, -25.372) -> (-3.5, -27.2764) centre (0, 0) ccw
  line L12 (-3.5, -27.2764) -> (-3.5, -19.5)
  arc A13 (-2.5, -18.5) -> (-3.5, -19.5) centre (-2.5, -19.5) ccw
  line L13 (-2.5, -18.5) -> (2.5, -18.5)
  arc A14 (3.5, -19.5) -> (2.5, -18.5) centre (2.5, -19.5) ccw
  line L14 (3.5, -19.5) -> (3.5, -27.2764)
  arc A15 (3.5, -27.2764) -> (10.6071, -25.372) centre (0, 0) ccw
  line L15 (10.6071, -25.372) -> (6.7189, -18.6375)
  arc A16 (7.0849, -17.2715) -> (6.7189, -18.6375) centre (7.5849, -18.1375) ccw
  line L16 (7.0849, -17.2715) -> (11.4151, -14.7715)
  arc A17 (12.7811, -15.1375) -> (11.4151, -14.7715) centre (11.9151, -15.6375) ccw
  line L17 (12.7811, -15.1375) -> (16.6693, -21.872)
  arc A18 (16.6693, -21.872) -> (21.872, -16.6693) centre (0, 0) ccw
  line L18 (21.872, -16.6693) -> (15.1375, -12.7811)
  arc A19 (14.7715, -11.4151) -> (15.1375, -12.7811) centre (15.6375, -11.9151) ccw
  line L19 (14.7715, -11.4151) -> (17.2715, -7.0849)
  arc A20 (18.6375, -6.7189) -> (17.2715, -7.0849) centre (18.1375, -7.5849) ccw
  line L20 (18.6375, -6.7189) -> (25.372, -10.6071)
  arc A21 (25.372, -10.6071) -> (27.2764, -3.5) centre (0, 0) ccw
  line L21 (27.2764, -3.5) -> (19.5, -3.5)
  arc A22 (18.5, -2.5) -> (19.5, -3.5) centre (19.5, -2.5) ccw
  line L22 (18.5, -2.5) -> (18.5, 2.5)
  arc A23 (19.5, 3.5) -> (18.5, 2.5) centre (19.5, 2.5) ccw
  line L23 (19.5, 3.5) -> (27.2764, 3.5)
  arc A24 (27.2764, 3.5) -> (25.372, 10.6071) centre (0, 0) ccw
  line L24 (25.372, 10.6071) -> (18.6375, 6.7189)
  arc A25 (17.2715, 7.0849) -> (18.6375, 6.7189) centre (18.1375, 7.5849) ccw
  line L25 (17.2715, 7.0849) -> (14.7715, 11.4151)
  arc A26 (15.1375, 12.7811) -> (14.7715, 11.4151) centre (15.6375, 11.9151) ccw
  line L26 (15.1375, 12.7811) -> (21.872, 16.6693)
  arc A27 (21.872, 16.6693) -> (16.6693, 21.872) centre (0, 0) ccw
  line L27 (16.6693, 21.872) -> (12.2811, 14.2715)
  line L28 (12.2811, 14.2715) -> (7.0849, 17.2715)
  arc A28 (6.7189, 18.6375) -> (7.0849, 17.2715) centre (7.5849, 18.1375) ccw
  line L29 (6.7189, 18.6375) -> (10.6071, 25.372)
  arc A29 (10.6071, 25.372) -> (3.5, 27.2764) centre (0, 0) ccw
  line L30 (3.5, 27.2764) -> (3.5, 19.5)
  arc A30 (2.5, 18.5) -> (3.5, 19.5) centre (2.5, 19.5) ccw
  line L31 (2.5, 18.5) -> (-2.5, 18.5)
  arc A31 (-3.5, 19.5) -> (-2.5, 18.5) centre (-2.5, 19.5) ccw
  line L32 (-3.5, 19.5) -> (-3.5, 27.2764)
  arc A32 (-3.5, 27.2764) -> (-10.6071, 25.372) centre (0, 0) ccw
  line L33 (-10.6071, 25.372) -> (-6.7189, 18.6375)
  arc A33 (-7.0849, 17.2715) -> (-6.7189, 18.6375) centre (-7.5849, 18.1375) ccw
  line L34 (-7.0849, 17.2715) -> (-11.4151, 14.7715)
  arc A34 (-12.7811, 15.1375) -> (-11.4151, 14.7715) centre (-11.9151, 15.6375) ccw
  line L35 (-12.7811, 15.1375) -> (-16.6693, 21.872)
  arc A35 (-16.6693, 21.872) -> (-21.872, 16.6693) centre (0, 0) ccw
  line L36 (-21.872, 16.6693) -> (-15.1375, 12.7811)
  arc A36 (-14.7715, 11.4151) -> (-15.1375, 12.7811) centre (-15.6375, 11.9151) ccw
  line L37 (-14.7715, 11.4151) -> (-17.2715, 7.0849)
  arc A37 (-18.6375, 6.7189) -> (-17.2715, 7.0849) centre (-18.1375, 7.5849) ccw
  line L38 (-18.6375, 6.7189) -> (-25.372, 10.6071)
  arc A38 (-25.372, 10.6071) -> (-27.2764, 3.5) centre (0, 0) ccw
  line L39 (-27.2764, 3.5) -> (-19.5, 3.5)
  arc A39 (-18.5, 2.5) -> (-19.5, 3.5) centre (-19.5, 2.5) ccw
  line L40 (-18.5, 2.5) -> (-18.5, -2.5)
  arc A40 (-19.5, -3.5) -> (-18.5, -2.5) centre (-19.5, -2.5) ccw
  line L41 (-19.5, -3.5) -> (-27.2764, -3.5)
  arc A41 (-27.2764, -3.5) -> (-25.372, -10.6071) centre (0, 0) ccw
  line L42 (-25.372, -10.6071) -> (-18.6375, -6.7189)
  arc A42 (-17.2715, -7.0849) -> (-18.6375, -6.7189) centre (-18.1375, -7.5849) ccw
  line L43 (-17.2715, -7.0849) -> (-14.7715, -11.4151)
  arc A43 (-15.1375, -12.7811) -> (-14.7715, -11.4151) centre (-15.6375, -11.9151) ccw
  line L44 (-15.1375, -12.7811) -> (-21.872, -16.6693)
  arc A44 (-21.872, -16.6693) -> (-16.6693, -21.872) centre (0, 0) ccw
  line L45 (-16.6693, -21.872) -> (-12.7811, -15.1375)
  arc A45 (-11.4151, -14.7715) -> (-12.7811, -15.1375) centre (-11.9151, -15.6375) ccw
  line L46 (-11.4151, -14.7715) -> (-7.0849, -17.2715)
  arc A46 (-6.7189, -18.6375) -> (-7.0849, -17.2715) centre (-7.5849, -18.1375) ccw
  line L47 (-6.7189, -18.6375) -> (-10.6071, -25.372)
  circle A47 centre (0, -16.7) radius 1.075
  circle A48 centre (14.4626, -8.35) radius 1.075
  circle A49 centre (14.4626, 8.35) radius 1.075
  circle A50 centre (0, 16.7) radius 1.075
  circle A51 centre (-14.4626, 8.35) radius 1.075
  circle A52 centre (-14.4626, -8.35) radius 1.075
  dimension "d33" = 2.15
  dimension "d35" = 360
  measures "d33" diameter of A47
extrude "押し出し7" cut sketch "スケッチ10" against normal blind 18 contours A47 | A48 | A49 | A50 | A51 | A52
